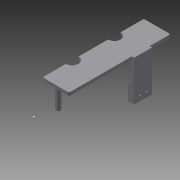
# Autodesk Inventor part: Latch
Saved by Autodesk Inventor 2015 SP2 (Build 190223200, 223)
## iProperties
Created: 2016-08-31
Part Number: Latch
Material: Generic
Document SubType Name: Modeling
Designer: jm799
Density: 1 g/cm^3
Appearance: Default
Author: jm799
Autodesk Inventor part; units mm, degrees
ref_plane "YZ Plane" through (0, 0, 0) normal (1, 0, 0) x (0, 1, 0)
ref_plane "XZ Plane" through (0, 0, 0) normal (0, 1, 0) x (-1, 0, 0)
ref_plane "XY Plane" through (0, 0, 0) normal (0, 0, 1) x (1, 0, 0)
sketch "Sketch7" plane through (0, 0, 0) normal (0, 1, 0) x (-1, 0, 0)
  line L0 (13.5789, -22.6329) -> (-3.4211, -22.6329)
  line L1 (-3.4211, -22.6329) -> (-3.4211, -87.6329)
  line L2 (-3.4211, -87.6329) -> (13.5789, -87.6329)
  line L3 (13.5789, -87.6329) -> (13.5789, -22.6329)
  point P0 (0, 0)
  dimension "d16" = 65
  dimension "d17" = 17
  constraints: 8 end point, 2 parallel, 1 horizontal, 1 perpendicular
  measures "d16" distance of L0.end L1.end
  measures "d17" distance of L0.start L0.end
extrude "Extrusion4" add sketch "Sketch7" along normal blind 2
fillet "Fillet1" radius 1 4 edges at (3.4211, 1, -22.6329) (-13.5789, 1, -22.6329) (3.4211, 1, -87.6329) (-13.5789, 1, -87.6329)
sketch "Sketch15" plane through (0, 0, 0) normal (0, -1, 0) x (1, 0, 0)
  line L0 (-13.5789, -86.6329) -> (-13.5789, -23.6329) projected
  line L1 (-13.5789, -55.1329) -> (3.4211, -55.1329)
  line L2 (3.4211, -23.6329) -> (3.4211, -86.6329) projected
  line L3 (-13.5789, -55.1329) -> (-13.5789, -68.6329)
  circle A0 centre (-13.5789, -68.6329) radius 4
  circle A1 centre (-13.5789, -41.6329) radius 4
  point P0 (0, 0)
  dimension "d46" = 13.5
  dimension "d47" = 8
  constraints: 4 end point, 2 centre point, 2 midpoint, 1 coincident, 1 point on line, 1 symmetric about line, 1 other
  measures "d46" distance of L1.start L3.end
  measures "d47" diameter of A0
extrude "Extrusion8" cut sketch "Sketch15" against normal blind 5
sketch "Sketch16" plane through (0, 0, 0) normal (0, -1, 0) x (1, 0, 0)
  arc A0 (-13.5789, -72.6329) -> (-13.5789, -64.6329) centre (-13.5789, -68.6329) ccw projected
  line L0 (-13.5789, -68.6329) -> (-7.7855, -83.2432)
  line L1 (-13.5789, -68.6329) -> (2.1381, -68.6329) construction
  circle A1 centre (-7.7855, -83.2432) radius 1.5
  line L2 (-13.5789, -64.6329) -> (-13.5789, -45.6329) construction
  line L3 (-13.5789, -55.1329) -> (3.4211, -55.1329) construction
  line L4 (3.4211, -23.6329) -> (3.4211, -86.6329) construction
  line L5 (-13.5789, -41.6329) -> (-7.7855, -27.0227)
  circle A2 centre (-7.7855, -27.0227) radius 1.5
  circle A3 centre (-7.7855, -83.2432) radius 2
  circle A4 centre (-7.7855, -27.0227) radius 2
  point P0 (0, 0)
  dimension "d50" = 15.717
  dimension "d51" = 68.37
  dimension "d52" = 3
  dimension "d55" = 4
  dimension "d56" = 4
  constraints: 8 end point, 4 centre point, 4 coincident, 3 symmetric about line, 2 midpoint, 1 equal length, 1 horizontal, 1 other
  measures "d50" distance of L0.start L0.end
  measures "d51" angle of L0 L1
  measures "d52" diameter of A1
  measures "d55" diameter of A3
  measures "d56" diameter of A4
extrude "Extrusion9" add sketch "Sketch16" along normal blind 15 contours A1 | A2
sketch "Sketch17" plane through (0, 2, 0) normal (0, 1, 0) x (1, 0, 0)
  line L0 (-12.5789, 22.6329) -> (2.4211, 22.6329) construction
  line L1 (0, 22.6329) -> (0, 87.6329) construction
  line L2 (2.4211, 87.6329) -> (-12.5789, 87.6329) construction
  arc A0 (-13.5789, 64.6329) -> (-13.5789, 72.6329) centre (-13.5789, 68.6329) ccw construction
  line L3 (-13.5789, 68.6329) -> (3.4211, 68.6329) construction
  line L4 (3.4211, 23.6329) -> (3.4211, 86.6329) construction
  line L5 (-9.5789, 62.8384) -> (-9.5789, 74.4274) construction
  point P0 (0, 0)
  point P1 (-9.5789, 68.6329)
  dimension "d57" = 11.589
  constraints: 6 end point, 3 point on line, 2 vertical, 1 midpoint, 1 perpendicular, 1 point on circle
  measures "d57" distance of L5.start L5.end
sketch "Sketch25" plane through (0, 2, 0) normal (0, 1, 0) x (1, 0, 0)
  line L0 (3.4211, 23.6329) -> (3.4211, 86.6329) projected
  arc A0 (-13.5789, 64.6329) -> (-13.5789, 72.6329) centre (-13.5789, 68.6329) ccw projected
  point P0 (0, 0)
sketch "Sketch27" plane through (3.4211, 0, -86.6329) normal (1, 0, 0) x (0, 0, -1)
  line L0 (-63, 2) -> (0, 2) projected
  line L1 (-23.7493, 0) -> (-12.2507, 0)
  line L2 (-12.2507, 0) -> (-12.2507, 2)
  line L3 (-12.2507, 2) -> (-23.7493, 2)
  line L4 (-23.7493, 2) -> (-23.7493, 0)
  point P0 (-86.6329, 0)
  constraints: 8 end point, 2 parallel, 1 horizontal, 1 perpendicular, 1 point on line
extrude "Extrusion16" add sketch "Sketch27" along normal blind 1.5
sketch "Sketch28" plane through (0, 0, 0) normal (0, -1, 0) x (1, 0, 0)
  line L0 (4.9211, -74.3823) -> (3.4211, -74.3823)
  line L1 (3.4211, -74.3823) -> (3.4211, -62.8836)
  line L2 (3.4211, -62.8836) -> (4.9211, -62.8836)
  line L3 (4.9211, -62.8836) -> (4.9211, -74.3823)
  point P0 (0, 0)
  constraints: 8 end point, 2 parallel, 1 horizontal, 1 perpendicular
extrude "Extrusion17" add sketch "Sketch28" along normal blind 24
sketch "Sketch29" plane through (4.9211, 0, -86.6329) normal (1, 0, 0) x (0, 0, -1)
  line L0 (-22, 2) -> (-14, 2) construction
  line L1 (-18, 2) -> (-18, -24) construction
  line L2 (-23.7493, -24) -> (-12.2507, -24) construction
  circle A0 centre (-20.1722, -20.5985) radius 0.5
  circle A1 centre (-15.8278, -20.5985) radius 0.5
  point P0 (-86.6329, 0)
  dimension "d97" = 1
  constraints: 2 centre point, 2 end point, 2 midpoint
  measures "d97" diameter of A0
hole "Hole4" at (4.9211, -20.5985, -66.4608) at (4.9211, -20.5985, -70.8051) direction (-1, 0, 0) diameter 1 end through all
sketch "Sketch31" plane through (4.9211, 2, -74.3823) normal (0, 0, -1) x (-1, 0, 0)
  point P0 (4.9211, -2)
sketch "Sketch35" plane through (4.9211, 2, -74.3823) normal (0, 0, -1) x (-1, 0, 0)
  point P0 (4.9211, -2)
sketch "Sketch36" plane through (4.9211, 2, -74.3823) normal (0, 0, -1) x (-1, 0, 0)
  line L0 (1.5, -26) -> (1.5, -14)
  line L1 (1.5, -2) -> (1.5, -26) projected
  line L2 (1.5, -14) -> (4.0015, -16.5015)
  line L3 (1.5, -14) -> (5.0376, -14) construction
  line L4 (4.0015, -16.5015) -> (1.5, -16.5015)
  point P0 (4.9211, -2)
  dimension "d111" = 12
  dimension "d112" = 45
  constraints: 8 end point, 1 equal length, 1 horizontal, 1 midpoint, 1 perpendicular, 1 point on line
  measures "d111" distance of L0.start L0.end
  measures "d112" angle of L2 L3
extrude "Extrusion21" add sketch "Sketch36" against normal blind 11.499
sketch "Sketch38" plane through (4.9211, 2, -74.3823) normal (0, 0, -1) x (-1, 0, 0)
  line L0 (4.0015, -16.5015) -> (4.0015, -26)
  line L1 (4.0015, -26) -> (1.5, -26)
  line L2 (4.0015, -16.5015) -> (1.5, -16.5015)
  line L3 (1.5, -16.5015) -> (4.0015, -16.5015) projected
  line L4 (1.5, -16.5015) -> (1.5, -26)
  point P0 (4.9211, -2)
  constraints: 8 end point, 2 perpendicular, 1 collinear, 1 vertical
sketch "Sketch39" plane through (3.4211, 2, -62.8836) normal (0, 0, 1) x (1, 0, 0)
  line L0 (-2.5015, -16.5015) -> (-2.5015, -26)
  line L1 (-2.5015, -26) -> (0, -26)
  line L2 (0, -26) -> (1.5, -26) projected
  line L3 (-2.5015, -16.5015) -> (0, -16.5015)
  line L4 (-2.5015, -16.5015) -> (0, -16.5015) projected
  line L5 (0, -16.5015) -> (0, -26)
  line L6 (0, -16.5015) -> (0, -26) projected
  point P0 (-3.4211, -2)
  constraints: 8 end point, 3 collinear, 1 vertical
extrude "Extrusion22" add sketch "Sketch38" against normal blind 1
extrude "Extrusion23" add sketch "Sketch39" against normal blind 1
sketch "Sketch40" plane through (0, -24, 0) normal (0, -1, 0) x (1, 0, 0)
  line L0 (0.9196, -63.8836) -> (0.9196, -73.3823)
  line L1 (0.9196, -73.3823) -> (3.4211, -73.3823)
  line L2 (3.4211, -74.3823) -> (3.4211, -62.8836) projected
  line L3 (3.4211, -73.3823) -> (3.4211, -63.8836)
  line L4 (3.4211, -63.8836) -> (0.9196, -63.8836)
  line L5 (3.4211, -63.8836) -> (0.9196, -63.8836) projected
  point P0 (0, 0)
  constraints: 8 end point, 1 collinear, 1 perpendicular, 1 point on line, 1 vertical
extrude "Extrusion24" add sketch "Sketch40" against normal blind 0.5
sketch "Sketch41" plane through (3.4211, -14.5015, -73.3823) normal (-1, 0, 0) x (0, 0, 1)
  point P0 (73.3823, 14.5015)
body "Solid4"
